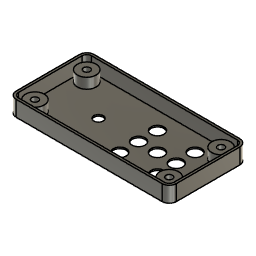
EDiceTop (Autodesk Fusion 360 design; units mm, degrees)
Autodesk Fusion 360 part; units mm, degrees
note: some values were not read from the file. Set by a fixed rule: which sketch regions a step uses.
sketch "Skizze1" plane through (0, 0, 0) normal (0, 0, 1) x (1, 0, 0)
  line L0 (1.5, 0) -> (69.5, 0)
  line L1 (69.5, 0) -> (69.5, 16.5)
  line L2 (69.5, 16.5) -> (1.5, 16.5)
  line L3 (1.5, 16.5) -> (1.5, 0)
  dimension "d1" = 68
  dimension "d2" = 16.5
  constraint horizontal L0
  constraint vertical L1
  constraint horizontal L2
  constraint vertical L3
  measures "d1" distance of L0.start L0.end
  measures "d2" distance of L0.end L1.end
extrude "Extrusion1" add sketch "Skizze1" along normal blind 0.6
sketch "Skizze2" plane through (0, 0, 0.6) normal (0, 0, 1) x (-1, 0, 0)
  line L0 (-1.5, -16.5) -> (-1.5, 0)
  line L1 (-1.5, 0) -> (-69.5, 0)
  line L2 (-69.5, 0) -> (-69.5, -16.5)
  line L3 (-69.5, -16.5) -> (-1.5, -16.5)
  line L4 (-1.5, 0) -> (-1.5, -16.5)
  line L5 (-1.5, -16.5) -> (-69.5, -16.5)
  line L6 (-69.5, -16.5) -> (-69.5, 0)
  line L7 (-69.5, 0) -> (-68.5, 0)
  line L8 (-68.5, 0) -> (-68.5, -15.5)
  line L9 (-68.5, -15.5) -> (-2.5, -15.5)
  line L10 (-2.5, -15.5) -> (-2.5, 0)
  line L11 (-2.5, 0) -> (-1.5, 0)
  dimension "d5" = 1
  dimension "d6" = 1
  dimension "d7" = 1
  constraint coincident L0.end L1.start
  constraint coincident L0.start L3.end
  constraint coincident L2.end L3.start
  constraint coincident L1.end L2.start
  constraint coincident L1 L7.end
  constraint perpendicular L6 L7
  constraint perpendicular L1 L8
  constraint perpendicular L8 L9
  constraint coincident L1 L10.end
  constraint perpendicular L1 L10
  measures "d5" distance of L0.end L10.end
  measures "d6" distance of L1.end L7.end
  measures "d7" vertical distance of L2.end L8.end
extrude "Extrusion2" add sketch "Skizze2" along normal blind 6 contours L0 L1 L2 L3 L4 L5 L6 L7 L8 L9 L10 L11
fillet "Abrundung1" radius 2 2 edges at (2.5, 15.5, 3.6) (68.5, 15.5, 3.6)
fillet "Abrundung2" radius 3 2 edges at (69.5, 16.5, 3.3) (1.5, 16.5, 3.3)
sketch "Skizze3" plane through (0, 0, 0.6) normal (0, 0, 1) x (-1, 0, 0)
  arc A0 (-68.5, -13.5) -> (-66.5, -15.5) centre (-66.5, -13.5) ccw
  line L0 (-66.5, -15.5) -> (-4.5, -15.5)
  arc A1 (-4.5, -15.5) -> (-2.5, -13.5) centre (-4.5, -13.5) ccw
  line L1 (-2.5, -13.5) -> (-2.5, 0)
  line L2 (-2.5, 0) -> (-68.5, 0)
  line L3 (-68.5, 0) -> (-68.5, -13.5)
  circle A2 centre (-64, -11) radius 4
  circle A3 centre (-7, -11) radius 4
  dimension "d14" = 8
  dimension "d15" = 8
  dimension "d16" = 57
  dimension "d17" = 11
  dimension "d18" = 7
  dimension "d19" = 11
  measures "d14" diameter of A3
  measures "d15" diameter of A2
  measures "d16" distance of A2.centre A3.centre
  measures "d17" distance of L2 A2.centre
  measures "d18" horizontal distance of origin A3.centre
  measures "d19" vertical distance of origin A3.centre
extrude "Extrusion3" add sketch "Skizze3" along normal blind 4.4 contours A2 | A3
sketch "Skizze4" plane through (0, 0, 5) normal (0, 0, 1) x (-1, 0, 0)
  circle A0 centre (-7, -11) radius 4
  circle A1 centre (-64, -11) radius 4
  point P0 (-7, -11)
  point P1 (-64, -11)
  constraint coincident P0 A0.centre
  constraint coincident P1 A1.centre
hole "Bohrung1" at (7, 11, 5) at (64, 11, 5) direction (0, 0, -1) diameter 2.8 depth 4 tip angle 180
sketch "Skizze5" plane through (0, 0, 0.6) normal (0, 0, 1) x (-1, 0, 0)
  circle A0 centre (-64, -11) radius 4
  circle A1 centre (-7, -11) radius 4
  arc A2 (-68.5, -13.5) -> (-66.5, -15.5) centre (-66.5, -13.5) ccw
  line L0 (-66.5, -15.5) -> (-4.5, -15.5)
  arc A3 (-4.5, -15.5) -> (-2.5, -13.5) centre (-4.5, -13.5) ccw
  line L1 (-2.5, -13.5) -> (-2.5, 0)
  line L2 (-2.5, 0) -> (-68.5, 0)
  line L3 (-68.5, 0) -> (-68.5, -13.5)
  circle A4 centre (-48, 0) radius 2.75
  circle A5 centre (-56, 0) radius 2.75
  circle A6 centre (-56, -8) radius 2.75
  circle A7 centre (-40, -8) radius 2.75
  circle A8 centre (-40, 0) radius 2.75
  circle A9 centre (-23, 0) radius 2
  dimension "d25" = 4
  dimension "d26" = 5.5
  dimension "d27" = 5.5
  dimension "d28" = 5.5
  dimension "d29" = 5.5
  dimension "d30" = 5.5
  dimension "d31" = 8
  dimension "d32" = 8
  dimension "d33" = 8
  dimension "d34" = 8
  dimension "d36" = 48
  dimension "d37" = 8
  dimension "d38" = 8
  dimension "d43" = 17
  constraint coincident L2 A4.centre
  constraint coincident L2 A5.centre
  constraint coincident L2 A8.centre
  constraint coincident L2 A9.centre
  measures "d25" diameter of A9
  measures "d26" diameter of A6
  measures "d27" diameter of A5
  measures "d28" diameter of A4
  measures "d29" diameter of A8
  measures "d30" diameter of A7
  measures "d31" distance of A4.centre A8.centre
  measures "d32" distance of A4.centre A5.centre
  measures "d33" horizontal distance of A4.centre A6.centre
  measures "d34" horizontal distance of A4.centre A7.centre
  measures "d36" distance of origin A4.centre
  measures "d37" distance of A7.centre A8.centre
  measures "d38" distance of A5.centre A6.centre
  measures "d43" distance of A8.centre A9.centre
extrude "Extrusion4" cut sketch "Skizze5" against normal blind 5 contours L2 A5 | L2 A4 | L2 A9 | L2 A8 | A6 | A7 picked at (-55.1334, -0.6679) picked at (-47.1334, -0.6679) picked at (-23.6445, -0.2959) picked at (-39.1334, -0.6679)
mirror "Spiegeln1" about plane through (0, 0, 0) normal (0, 1, 0) of bodies 1 merged
equation "d20 = 6 mm - 1.6 mm"
